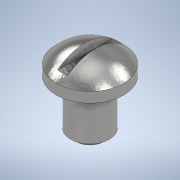
# Autodesk Inventor part: Pieza 1 KAS
Saved by Autodesk Inventor 2021 (Build 250183000, 183)
## iProperties
Created: 2020-10-13
Part Number: Pieza 1 KAS
Material: Steel, Galvanized
Document SubType Name: Modeling
Designer: The Godkiller
Density: 7.85 g/cm^3
Appearance: Galvanized
Author: The Godkiller
Autodesk Inventor part; units mm, degrees
ref_plane "YZ Plane" through (0, 0, 0) normal (1, 0, 0) x (0, 1, 0)
ref_plane "XZ Plane" through (0, 0, 0) normal (0, 1, 0) x (-1, 0, 0)
ref_plane "XY Plane" through (0, 0, 0) normal (0, 0, 1) x (1, 0, 0)
sketch "Sketch1" plane through (0, 0, 0) normal (0, 1, 0) x (-1, 0, 0)
  circle A0 centre (0, 0) radius 2.875
  dimension "d0" = 5.75
  constraints: 1 centre point, 1 coincident
  measures "d0" diameter of A0
extrude "Extrusion1" add sketch "Sketch1" along normal mid plane 6.75
sketch "Sketch2" plane through (0, -3.375, 0) normal (0, -1, 0) x (1, 0, 0)
  circle A0 centre (0, 0) radius 2
  dimension "d3" = 4
  constraints: 1 centre point, 1 coincident
  measures "d3" diameter of A0
extrude "Extrusion2" add sketch "Sketch2" along normal blind 0.75
sketch "Sketch3" plane through (0, 3.375, 0) normal (0, 1, 0) x (1, 0, 0)
  circle A0 centre (0, 0) radius 5
  dimension "d6" = 10
  constraints: 1 centre point, 1 coincident
  measures "d6" diameter of A0
extrude "Extrusion3" add sketch "Sketch3" along normal blind 1.5
sketch "Sketch5" plane through (0, 0, 0) normal (0, 0, 1) x (1, 0, 0)
  line L0 (5, 4.875) -> (-5, 4.875) projected
  line L1 (0, 4.875) -> (0, 7.225)
  line L2 (0, 4.875) -> (5, 4.875)
  arc A0 (5, 4.875) -> (0, 7.225) centre (-0.0027, 0.725) ccw
  line L3 (0, 4.875) -> (0, 12.9944) construction
  point P0 (0, 0)
  dimension "d9" = 2.35
  dimension "d10" = 6.5
  constraints: 6 end point, 2 point on circle, 2 vertical, 1 centre point, 1 horizontal, 1 midpoint
  measures "d9" distance of L1.start L1.end
  measures "d10" radius of A0
revolve "Revolution1" add sketch "Sketch5" angle 360 about axis through (0, 4.875, 0) along (0, 1, 0)
sketch "Sketch6" plane through (0, 0, 0) normal (0, 0, 1) x (1, 0, 0)
  line L0 (5, 4.875) -> (-5, 4.875) projected
  line L1 (0, 5.755) -> (0.75, 5.755)
  line L2 (0.75, 5.755) -> (0.75, 8.519)
  line L3 (0.75, 8.519) -> (-0.75, 8.519)
  line L4 (-0.75, 8.519) -> (-0.75, 5.755)
  line L5 (-0.75, 5.755) -> (0, 5.755)
  point P0 (0, 0)
  dimension "d13" = 0.75
  dimension "d14" = 1.5
  constraints: 10 end point, 4 perpendicular, 1 horizontal, 1 point on line
  measures "d13" distance of L1.start L1.end
  measures "d14" distance of L2.end L3.end
extrude "Extrusion4" cut sketch "Sketch6" against normal mid plane 15
body "Solid1"
